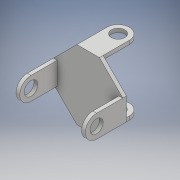
# Autodesk Inventor part: COXA2
Saved by Autodesk Inventor 2017 (Build 210142000, 142)
## iProperties
Created: 2017-09-24
Part Number: COXA2
Material: Generic
Document SubType Name: Modeling
Designer: Alexander Miller
Density: 1 g/cm^3
Appearance: Default
Author: Alexander Miller
Autodesk Inventor part; units mm, degrees
ref_plane "YZ Plane" through (0, 0, 0) normal (1, 0, 0) x (0, 1, 0)
ref_plane "XZ Plane" through (0, 0, 0) normal (0, 1, 0) x (-1, 0, 0)
ref_plane "XY Plane" through (0, 0, 0) normal (0, 0, 1) x (1, 0, 0)
sketch "Sketch1" plane through (0, 0, 0) normal (0, 1, 0) x (-1, 0, 0)
  line L0 (18.5, 6) -> (-18.5, 6) construction
  line L1 (-18.5, 6) -> (-18.5, -6)
  line L2 (-18.5, -6) -> (18.5, -6) construction
  line L3 (18.5, -6) -> (18.5, 6)
  line L4 (6, 18.5) -> (-6, 18.5)
  line L5 (-6, 18.5) -> (-6, -18.5) construction
  line L6 (-6, -18.5) -> (6, -18.5)
  line L7 (6, -18.5) -> (6, 18.5) construction
  line L8 (18.5, 6) -> (6, 18.5)
  line L9 (-6, 18.5) -> (-18.5, 6)
  line L10 (-18.5, -6) -> (-6, -18.5)
  line L11 (6, -18.5) -> (18.5, -6)
  point P0 (0, 0)
  point P1 (0, -6)
  point P2 (18.5, 0)
  point P3 (0, 18.5)
  point P4 (6, 0)
  dimension "d0" = 37
  dimension "d1" = 12
  constraints: 24 end point, 7 perpendicular, 4 midpoint, 4 parallel, 2 horizontal, 2 horizontal alignment, 2 vertical alignment
  measures "d0" distance of L1.end L2.end
  measures "d1" distance of L2.end L0.start
extrude "Extrusion1" add sketch "Sketch1" along normal blind 2
sketch "Sketch2" plane through (0, 0, 0) normal (0, -1, 0) x (1, 0, 0)
  line L0 (-18.5, 6) -> (-16.5, 6)
  line L1 (-16.5, 6) -> (-16.5, -6)
  line L2 (-16.5, -6) -> (-18.5, -6)
  line L3 (-18.5, -6) -> (-18.5, 6)
  line L4 (16.5, 6) -> (18.5, 6)
  line L5 (18.5, 6) -> (18.5, -6)
  line L6 (18.5, -6) -> (16.5, -6)
  line L7 (16.5, -6) -> (16.5, 6)
  line L8 (-18.5, 6) -> (-18.5, -6) projected
  line L9 (18.5, -6) -> (18.5, 6) projected
  point P0 (0, 0)
  point P1 (17.5, 6)
  point P2 (17.5, -6)
  point P3 (-17.5, -6)
  point P4 (-17.5, 6)
  dimension "d4" = 2
  constraints: 16 end point, 4 horizontal alignment, 4 midpoint, 4 parallel, 3 collinear, 2 horizontal, 2 perpendicular
  measures "d4" distance of L0.start L0.end
extrude "Extrusion2" add sketch "Sketch2" along normal blind 20
full round fillet "Fillet1" first side at (-17.8333, -6.6667, 6) centre faces at (-17.1667, -20, -2) second side at (-17.1667, -6.6667, -6)
full round fillet "Fillet2" first side at (17.8333, -6.6667, -6) centre faces at (17.1667, -20, 2) second side at (17.1667, -6.6667, 6)
sketch "Sketch3" plane through (0, 2, 0) normal (0, 1, 0) x (1, 0, 0)
  line L0 (-6, -18.5) -> (6, -18.5)
  line L1 (6, -18.5) -> (6, -16.5)
  line L2 (6, -16.5) -> (-6, -16.5)
  line L3 (-6, -16.5) -> (-6, -18.5)
  line L4 (-6, 16.5) -> (6, 16.5)
  line L5 (6, 16.5) -> (6, 18.5)
  line L6 (6, 18.5) -> (-6, 18.5)
  line L7 (-6, 18.5) -> (-6, 16.5)
  line L8 (-6, -18.5) -> (6, -18.5) projected
  line L9 (6, 18.5) -> (-6, 18.5) projected
  point P0 (0, 0)
  point P1 (-6, -17.5)
  point P2 (6, -17.5)
  point P3 (-6, 17.5)
  dimension "d7" = 2
  constraints: 16 end point, 4 parallel, 3 collinear, 3 midpoint, 3 vertical alignment, 2 horizontal, 2 perpendicular, 1 point on line
  measures "d7" distance of L2.end L0.start
extrude "Extrusion3" add sketch "Sketch3" along normal blind 20
full round fillet "Fillet3" first side at (6, 8.6667, 17.8333) centre faces at (-2, 22, 17.1667) second side at (-6, 8.6667, 17.1667)
full round fillet "Fillet4" first side at (-6, 15.3333, -17.1667) centre faces at (2, 22, -17.1667) second side at (6, 15.3333, -17.8333)
sketch "Sketch4" plane through (18.5, 2, 6) normal (1, 0, 0) x (0, 0, -1)
  circle A0 centre (6, -16) radius 3.5
  arc A1 (0, -16) -> (12, -16) centre (6, -16) ccw projected
  point P0 (6, -2)
  dimension "d10" = 7
  constraints: 1 centre point, 1 concentric
  measures "d10" diameter of A0
extrude "Extrusion4" cut sketch "Sketch4" against normal up to surface (2 mm away)
sketch "Sketch5" plane through (6, 0, -18.5) normal (0, 0, -1) x (-1, 0, 0)
  circle A0 centre (6, 16) radius 3.5
  arc A1 (12, 16) -> (0, 16) centre (6, 16) ccw projected
  point P0 (6, 0)
  dimension "d13" = 7
  constraints: 1 centre point, 1 concentric
  measures "d13" diameter of A0
extrude "Extrusion5" cut sketch "Sketch5" against normal up to surface (2 mm away)
sketch "Sketch6" plane through (-18.5, 2, -6) normal (-1, 0, 0) x (0, 0, 1)
  circle A0 centre (6, -16) radius 3.625
  arc A1 (0, -16) -> (12, -16) centre (6, -16) ccw projected
  point P0 (6, -2)
  dimension "d16" = 7.25
  constraints: 1 centre point, 1 concentric
  measures "d16" diameter of A0
extrude "Extrusion6" cut sketch "Sketch6" against normal up to surface (2 mm away)
sketch "Sketch7" plane through (-6, 0, 18.5) normal (0, 0, 1) x (1, 0, 0)
  circle A0 centre (6, 16) radius 3.625
  arc A1 (12, 16) -> (0, 16) centre (6, 16) ccw projected
  point P0 (6, 0)
  dimension "d19" = 7.25
  constraints: 1 centre point, 1 concentric
  measures "d19" diameter of A0
extrude "Extrusion7" cut sketch "Sketch7" against normal up to surface (2 mm away)
equation "\"d1\" = servo_B"
equation "\"d10\" = bearing_A"
equation "\"d13\" = bearing_A"
equation "\"d16\" = servo_hat_A"
equation "\"d19\" = servo_hat_A"
equation "\"servo_B\" = 12"
equation "\"bearing_A\" = 7"
equation "\"servo_hat_A\" = 7.25"
body "Solid1"
